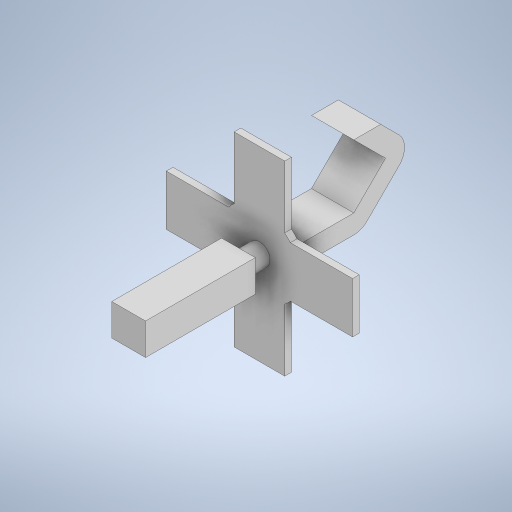
# Autodesk Inventor part: Pieza1
Saved by Autodesk Inventor 2023 (Build 270158000, 158)
## iProperties
Created: 2023-05-30
Part Number: Pieza1
Material: Genérico
Document SubType Name: Modeling
Designer: WIN10
Density: 1 g/cm^3
Appearance: Valor por defecto
Author: WIN10
Autodesk Inventor part; units mm, degrees
ref_plane "YZ Plane" through (0, 0, 0) normal (1, 0, 0) x (0, 1, 0)
ref_plane "XZ Plane" through (0, 0, 0) normal (0, 1, 0) x (-1, 0, 0)
ref_plane "XY Plane" through (0, 0, 0) normal (0, 0, 1) x (1, 0, 0)
sketch "Boceto1" plane through (0, 0, 0) normal (1, 0, 0) x (0, 1, 0)
  line L0 (0, 0) -> (0, 14.3) construction
  line L1 (0, 14.3) -> (-23.8, 14.3) construction
  line L2 (-23.8, 14.3) -> (-23.8, 38.1) construction
  line L3 (-23.8, 38.1) -> (0, 14.3)
  circle A0 centre (0, 14.3) radius 14.3 construction
  line L4 (-10.1116, 4.1884) -> (-23.8, 17.8767)
  arc A1 (-10.1116, 4.1884) -> (0, 0) centre (0, 14.3) ccw
  line L5 (23.8, 38.1) -> (0, 14.3)
  line L6 (10.1116, 4.1884) -> (23.8, 17.8767)
  arc A2 (0, 0) -> (10.1116, 4.1884) centre (0, 14.3) ccw
  line L7 (23.8, 38.1) -> (23.8, 17.8767)
  circle A3 centre (-23.8, 38.1) radius 14.3 construction
  line L8 (-23.8, 38.1) -> (-23.8, 88.1)
  line L9 (-23.8, 17.8767) -> (-33.9116, 27.9884)
  line L10 (-38.1, 38.1) -> (-38.1, 88.1)
  line L11 (-38.1, 88.1) -> (-23.8, 88.1)
  arc A4 (-38.1, 38.1) -> (-33.9116, 27.9884) centre (-23.8, 38.1) ccw
  dimension "d0" = 14.3
  dimension "d1" = 23.8
  dimension "d2" = 23.8
  dimension "d3" = 28.6
  dimension "d4" = 50
  dimension "d7" = 23.8
  dimension "d8" = 47.6
  dimension "d9" = 47.9583
  constraints: 24 end point, 10 point on circle, 5 centre point, 5 coincident, 4 parallel, 3 point on line, 3 symmetric about line, 3 tangent, 1 horizontal, 1 perpendicular
  measures "d0" distance of point (0, 0) L0.end
  measures "d1" distance of L0.end L1.end
  measures "d2" distance of L1.end L2.end
  measures "d3" diameter of A3
  measures "d4" distance of L8.start L8.end
  measures "d7" distance from line of point (0, 0) L7
  measures "d8" distance from line of point (-23.8, 38.1) L7
  measures "d9" distance from line of point (-23.8, 38.1) L6
extrude "Extrusión1" add sketch "Boceto1" along normal mid plane 31.8
sketch "Boceto2" plane through (-15.9, -38.1, 88.1) normal (0, 0, 1) x (1, 0, 0)
  line L0 (0, 14.3) -> (31.8, 14.3) construction
  line L1 (31.8, 0) -> (31.8, 4.1884) construction
  line L2 (0, 14.3) -> (31.8, 0) construction
  line L3 (15.9, 7.15) -> (-3.1, 7.15) construction
  line L4 (-3.1, 7.15) -> (-3.1, 77.15) construction
  line L5 (-3.1, 77.15) -> (15.9, 77.15) construction
  line L6 (15.9, 77.15) -> (15.9, 7.15) construction
  line L7 (15.9, 7.15) -> (-54.1, 7.15) construction
  line L8 (-54.1, 7.15) -> (-54.1, 26.15) construction
  line L9 (-54.1, 26.15) -> (15.9, 26.15) construction
  line L10 (15.9, 26.15) -> (15.9, 7.15) construction
  circle A0 centre (15.9, 7.15) radius 30 construction
  line L11 (15.9, 77.15) -> (-3.1, 77.15)
  line L12 (-3.1, 30.3664) -> (-3.1, 77.15)
  line L13 (-54.1, 7.15) -> (-54.1, 26.15)
  line L14 (-54.1, 26.15) -> (-7.3164, 26.15)
  arc A1 (-3.1, 30.3664) -> (-7.3164, 26.15) centre (15.9, 7.15) ccw
  line L15 (-54.1, -11.85) -> (-54.1, 7.15) construction
  line L16 (15.9, -11.85) -> (-54.1, -11.85) construction
  line L17 (-7.3164, -11.85) -> (-54.1, -11.85)
  line L18 (-54.1, 7.15) -> (-54.1, -11.85)
  line L19 (15.9, -62.85) -> (-3.1, -62.85) construction
  line L20 (15.9, -62.85) -> (-3.1, -62.85)
  line L21 (-3.1, -62.85) -> (-3.1, 7.15) construction
  line L22 (-3.1, -62.85) -> (-3.1, -16.0664)
  arc A2 (-7.3164, -11.85) -> (-3.1, -16.0664) centre (15.9, 7.15) ccw
  line L23 (34.9, -62.85) -> (15.9, -62.85) construction
  line L24 (34.9, 7.15) -> (34.9, -62.85) construction
  line L25 (34.9, -16.0664) -> (34.9, -62.85)
  line L26 (15.9, -62.85) -> (34.9, -62.85)
  line L27 (85.9, 7.15) -> (85.9, -11.85) construction
  line L28 (85.9, 7.15) -> (85.9, -11.85)
  line L29 (85.9, -11.85) -> (15.9, -11.85) construction
  line L30 (85.9, -11.85) -> (39.1164, -11.85)
  arc A3 (34.9, -16.0664) -> (39.1164, -11.85) centre (15.9, 7.15) ccw
  line L31 (85.9, 26.15) -> (85.9, 7.15) construction
  line L32 (15.9, 26.15) -> (85.9, 26.15) construction
  line L33 (39.1164, 26.15) -> (85.9, 26.15)
  line L34 (85.9, 7.15) -> (85.9, 26.15)
  line L35 (15.9, 77.15) -> (34.9, 77.15) construction
  line L36 (15.9, 77.15) -> (34.9, 77.15)
  line L37 (34.9, 77.15) -> (34.9, 7.15) construction
  line L38 (34.9, 77.15) -> (34.9, 30.3664)
  arc A4 (39.1164, 26.15) -> (34.9, 30.3664) centre (15.9, 7.15) ccw
  point P0 (15.9, 38.1)
  point P1 (-54.1, 7.15)
  point P2 (85.9, 7.15)
  dimension "d10" = 19
  dimension "d11" = 70
  dimension "d12" = 70
  dimension "d13" = 19
  dimension "d14" = 60
  dimension "d17" = 360
  constraints: 74 end point, 10 point on circle, 8 point on line, 6 equal length, 5 centre point, 4 coincident, 3 perpendicular, 2 horizontal, 1 midpoint, 71 other
  measures "d10" distance of L4.end L5.end
  measures "d11" distance of L3.end L4.end
  measures "d12" distance of L8.end L9.end
  measures "d13" distance of L7.end L8.end
  measures "d14" diameter of A0
extrude "Extrusión2" add sketch "Boceto2" along normal blind 5
sketch "Boceto3" plane through (-15.9, -38.1, 93.1) normal (0, 0, 1) x (1, 0, 0)
  arc A0 (39.1164, 26.15) -> (34.9, 30.3664) centre (15.9, 7.15) ccw projected
  circle A1 centre (15.9, 7.15) radius 7.9
  point P0 (15.9, 38.1)
  dimension "d21" = 15.8
  constraints: 1 centre point, 1 coincident
  measures "d21" diameter of A1
extrude "Extrusión3" add sketch "Boceto3" along normal blind 15.8
sketch "Boceto4" plane through (0, -30.95, 108.9) normal (0, 0, 1) x (1, 0, 0)
  line L0 (12.7, 11.9) -> (-12.7, 11.9)
  line L1 (-12.7, 11.9) -> (-12.7, -11.9)
  line L2 (-12.7, -11.9) -> (12.7, -11.9)
  line L3 (12.7, -11.9) -> (12.7, 11.9)
  circle A0 centre (0, 0) radius 7.9 projected
  point P0 (0, 30.95)
  point P1 (12.7, 0)
  point P2 (0, -11.9)
  dimension "d24" = 25.4
  dimension "d25" = 23.8
  constraints: 8 end point, 2 midpoint, 2 parallel, 1 horizontal, 1 horizontal alignment, 1 perpendicular, 1 vertical alignment
  measures "d24" distance of L0.start L0.end
  measures "d25" distance of L0.end L1.end
extrude "Extrusión4" add sketch "Boceto4" along normal blind 82.5 contours L3 L2 L1 L0 | A0
